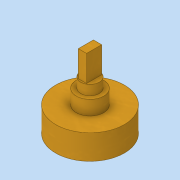
# Autodesk Inventor part: potentiometer
Saved by Autodesk Inventor 2017 (Build 210142000, 142)
## iProperties
Created: 2016-12-10
Part Number: potentiometer
Material: Brass, Soft Yellow, Welded
Document SubType Name: Modeling
Designer: techn
Density: 8.5 g/cm^3
Appearance: Weld - Brass
Author: techn
Autodesk Inventor part; units mm, degrees
ref_plane "YZ Plane" through (0, 0, 0) normal (1, 0, 0) x (0, 1, 0)
ref_plane "XZ Plane" through (0, 0, 0) normal (0, 1, 0) x (-1, 0, 0)
ref_plane "XY Plane" through (0, 0, 0) normal (0, 0, 1) x (1, 0, 0)
sketch "Sketch1" plane through (0, 0, 0) normal (0, 0, 1) x (1, 0, 0)
  line L0 (0, 0) -> (6.35, 0)
  line L1 (6.35, 0) -> (6.35, 4.572)
  line L2 (6.35, 4.572) -> (2.54, 4.572)
  line L3 (2.54, 4.572) -> (2.54, 7.239)
  line L4 (2.54, 7.239) -> (1.7272, 7.239)
  line L5 (1.7272, 7.239) -> (1.7272, 9.0678)
  line L6 (1.7272, 9.0678) -> (0, 9.0678)
  line L7 (0, 0) -> (0, 9.0678)
  dimension "d0" = 6.35
  dimension "d1" = 4.572
  dimension "d2" = 3.81
  dimension "d3" = 2.667
  dimension "d4" = 1.7272
  dimension "d5" = 1.8288
  constraints: 16 end point, 5 perpendicular, 1 horizontal, 1 parallel, 1 vertical
  measures "d0" distance of L0.start L0.end
  measures "d1" distance of L0.end L1.end
  measures "d2" distance of L1.end L2.end
  measures "d3" distance of L2.end L3.end
  measures "d4" horizontal distance of L0.start L4.end
  measures "d5" distance of L4.end L5.end
revolve "Revolution1" add sketch "Sketch1" angle 360 about axis through (0, 0, 0) along (0, 1, 0)
sketch "Sketch2" plane through (0, 9.0678, 0) normal (0, 1, 0) x (1, 0, 0)
  line L0 (-0.762, -1.397) -> (0.762, -1.397)
  line L1 (0.762, -1.397) -> (0.762, 1.397)
  line L2 (0.762, 1.397) -> (-0.762, 1.397)
  line L3 (-0.762, 1.397) -> (-0.762, -1.397)
  point P0 (0, 0)
  dimension "d7" = 2.794
  dimension "d8" = 1.524
  dimension "d9" = 1.397
  dimension "d10" = 0.762
  constraints: 8 end point, 2 parallel, 1 horizontal, 1 perpendicular
  measures "d7" distance of L2.end L0.start
  measures "d8" distance of L0.start L0.end
  measures "d9" distance from line of L2 point (0, 0)
  measures "d10" distance from line of L1 point (0, 0)
extrude "Extrusion1" add sketch "Sketch2" along normal blind 4.826
equation "\"d9\" = 0.5 * d7"
equation "\"d10\" = 0.5 * d8"
body "Solid1"
